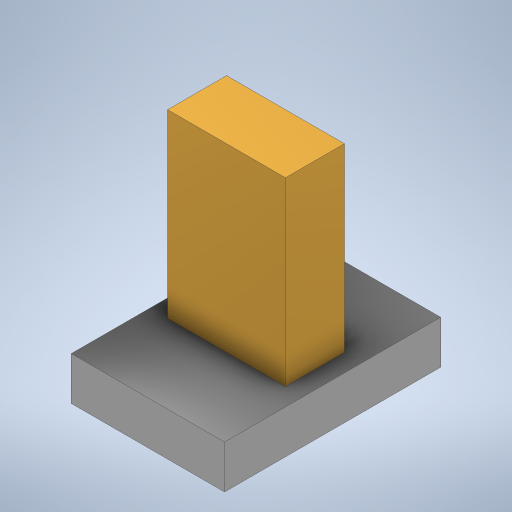
# Autodesk Inventor part: mirror
Saved by Autodesk Inventor 2023 (Build 270158000, 158)
## iProperties
Created: 2023-04-11
Part Number: mirror
Material: Generic
Document SubType Name: Modeling
Designer: Sam
Density: 1 g/cm^3
Appearance: Default
Author: Sam
Autodesk Inventor part; units mm, degrees
ref_plane "YZ Plane" through (0, 0, 0) normal (1, 0, 0) x (0, 1, 0)
ref_plane "XZ Plane" through (0, 0, 0) normal (0, 1, 0) x (-1, 0, 0)
ref_plane "XY Plane" through (0, 0, 0) normal (0, 0, 1) x (1, 0, 0)
sketch "Sketch1" plane through (0, 0, 0) normal (0, 1, 0) x (-1, 0, 0)
  line L0 (-4.953, 6.985) -> (4.953, 6.985)
  line L1 (4.953, 6.985) -> (4.953, -6.985)
  line L2 (4.953, -6.985) -> (-4.953, -6.985)
  line L3 (-4.953, -6.985) -> (-4.953, 6.985)
  line L4 (-4.953, 6.985) -> (4.953, -6.985) construction
  line L5 (4.953, 6.985) -> (-4.953, -6.985) construction
  point P0 (0, 0)
  dimension "d0" = 13.97
  dimension "d1" = 9.906
  constraints: 12 end point, 2 midpoint, 2 parallel, 1 horizontal, 1 perpendicular
  measures "d0" distance of L0.end L1.end
  measures "d1" distance of L0.start L0.end
extrude "Extrusion1" add sketch "Sketch1" along normal mid plane 2.794
sketch "Sketch2" plane through (0, 1.397, 0) normal (0, 1, 0) x (1, 0, 0)
  line L0 (3.81, -1.905) -> (-3.81, -1.905)
  line L1 (-3.81, -1.905) -> (-3.81, 1.905)
  line L2 (-3.81, 1.905) -> (3.81, 1.905)
  line L3 (3.81, 1.905) -> (3.81, -1.905)
  line L4 (3.81, -1.905) -> (-3.81, 1.905) construction
  line L5 (-3.81, -1.905) -> (3.81, 1.905) construction
  point P0 (0, 0)
  dimension "d4" = 3.81
  dimension "d5" = 7.62
  constraints: 12 end point, 2 midpoint, 2 parallel, 1 horizontal, 1 perpendicular
  measures "d4" distance of L0.end L1.end
  measures "d5" distance of L1.end L2.end
extrude "Extrusion2" add sketch "Sketch2" along normal blind 11.684
body "Solid1"
